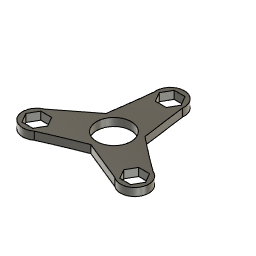
FIdget Spinner (Autodesk Fusion 360 design; units mm, degrees)
Autodesk Fusion 360 part; units mm, degrees
sketch "Sketch1" plane through (0, 0, 0) normal (0, 0, 1) x (1, 0, 0)
  circle A0 centre (0, 0) radius 11
  circle A1 centre (0, 0) radius 13.5
  circle A2 centre (0, 0) radius 45 construction
  circle A3 centre (-0.0744, 35.9127) radius 9
  arc A4 (-13.3245, 2.1699) -> (-8.9923, 34.7002) centre (-571.0597, 92.9983) ccw
  line L0 (8.8488, 34.7395) -> (13.3741, 1.8396)
  line L1 (-3.5385, 41.9127) -> (-7.0026, 35.9127)
  line L2 (-7.0026, 35.9127) -> (-3.5385, 29.9127)
  line L3 (-3.5385, 29.9127) -> (3.3897, 29.9127)
  line L4 (3.3897, 29.9127) -> (6.8538, 35.9127)
  line L5 (6.8538, 35.9127) -> (3.3897, 41.9127)
  line L6 (3.3897, 41.9127) -> (-3.5385, 41.9127)
  line L7 (-27.6, -24.0208) -> (-24.1359, -18.0208)
  line L8 (-34.5282, -24.0208) -> (-27.6, -24.0208)
  line L9 (-24.1359, -18.0208) -> (-27.6, -12.0208)
  circle A5 centre (-31.0641, -18.0208) radius 9
  line L10 (-34.5282, -12.0208) -> (-37.9923, -18.0208)
  arc A6 (4.783, -12.6243) -> (-25.5551, -25.1377) centre (204.991, -541.0514) ccw
  line L11 (-27.6, -12.0208) -> (-34.5282, -12.0208)
  line L12 (-34.5097, -9.7065) -> (-8.2801, 10.6625)
  line L13 (-37.9923, -18.0208) -> (-34.5282, -24.0208)
  line L14 (34.6026, -11.8919) -> (27.6744, -11.8919)
  line L15 (38.0667, -17.8919) -> (34.6026, -11.8919)
  line L16 (27.6744, -11.8919) -> (24.2103, -17.8919)
  circle A7 centre (31.1385, -17.8919) radius 9
  line L17 (27.6744, -23.8919) -> (34.6026, -23.8919)
  arc A8 (8.5414, 10.4544) -> (34.5474, -9.5625) centre (366.0688, 448.0531) ccw
  line L18 (24.2103, -17.8919) -> (27.6744, -23.8919)
  line L19 (25.6609, -25.0331) -> (-5.0939, -12.5021)
  line L20 (34.6026, -23.8919) -> (38.0667, -17.8919)
  point P0 (-0.0744, 35.9127)
  point P1 (-31.0641, -18.0208)
  point P2 (31.1385, -17.8919)
  dimension "d1" = 22
  dimension "d2" = 27
  dimension "d4" = 90
  dimension "d5" = 18
  dimension "d6" = 6
  dimension "d8" = 360
  constraint coincident A0.centre A1.centre
  constraint concentric A0 A2
  constraint tangent A1 A4
  constraint coincident A1 A4.start
  constraint coincident A3 A4.end
  constraint coincident A3 L0.start
  constraint coincident A1 L0.end
  constraint tangent A1 L0
  constraint coincident P0 A3.centre
  measures "d1" diameter of A0
  measures "d2" diameter of A1
  measures "d4" diameter of A2
  measures "d5" diameter of A3
  measures "d6" distance of P0 L6
extrude "Extrude1" add sketch "Sketch1" along normal blind 5
